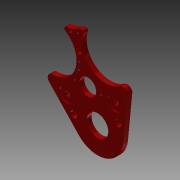
# Autodesk Inventor part: OutlineSketch1
Saved by Autodesk Inventor 2013 (Build 170138000, 138)
## iProperties
Created: 2013-06-03
Part Number: OutlineSketch1
Material: Aluminum 6061
Document SubType Name: Modeling
Designer: mvarma
Density: 2.71 g/cm^3
Mass: 149.846 g
Surface Area: 274.597 cm^2
Volume: 55.2937 cm^3
Author: mvarma
Autodesk Inventor part; units mm, degrees
ref_plane "YZ Plane" through (0, 0, 0) normal (1, 0, 0) x (0, 1, 0)
ref_plane "XZ Plane" through (0, 0, 0) normal (0, 1, 0) x (-1, 0, 0)
ref_plane "XY Plane" through (0, 0, 0) normal (0, 0, 1) x (1, 0, 0)
sketch "Sketch1" plane through (0, 0, 0) normal (0, 0, 1) x (1, 0, 0)
  line L0 (0, 0) -> (304.8, 0) construction
  line L1 (304.8, 0) -> (304.8, 50.8) construction
  line L2 (304.8, 50.8) -> (0, 50.8) construction
  line L3 (0, 50.8) -> (0, 0) construction
  circle A0 centre (152.4, 23.8125) radius 14.2875
  arc A1 (186.526662, 20.469591) -> (127.726757, 0) centre (152.4, 23.8125) ccw
  circle A2 centre (152.4, 23.8125) radius 26.035 construction
  line L4 (152.4, 23.8125) -> (139.519977, 61.741013) construction
  circle A3 centre (139.519977, 61.741013) radius 9.525 construction
  circle A4 centre (139.519977, 61.741013) radius 17.78 construction
  circle A5 centre (91.561866, 85.09) radius 31.75 construction
  arc A6 (133.1868, 119.400632) -> (182.101149, 83.849872) centre (163.342398, 109.465722) ccw
  circle A7 centre (109.531215, 150.050573) radius 31.75 construction
  line L5 (0, 50.8) -> (0, 53.34) construction
  line L6 (0, 53.34) -> (304.8, 53.34) construction
  line L7 (304.8, 53.34) -> (304.8, 50.8) construction
  circle A8 centre (139.519977, 61.741013) radius 21.59 construction
  circle A9 centre (152.4, 23.8125) radius 46.99 construction
  circle A10 centre (152.4, 23.8125) radius 50.8 construction
  arc A11 (86.386473, 79.456368) -> (92.43632, 92.689857) centre (91.561866, 85.09) ccw construction
  circle A12 centre (163.342398, 109.465722) radius 7.65 construction
  arc A13 (116.774938, 152.510446) -> (102.287492, 147.5907) centre (109.531215, 150.050573) ccw construction
  circle A14 centre (139.519977, 61.741013) radius 22.9 construction
  line L8 (86.386473, 79.456368) -> (124.027623, 44.87694) construction
  line L9 (170.878164, 108.148633) -> (162.078023, 57.798354) construction
  line L10 (92.43632, 92.689857) -> (91.561866, 85.09) construction
  line L11 (91.561866, 85.09) -> (86.386473, 79.456368) construction
  circle A15 centre (127.673753, 96.62524) radius 3.175 construction
  circle A16 centre (127.673753, 96.62524) radius 7.9375 construction
  line L12 (92.43632, 92.689857) -> (126.766436, 88.739767) construction
  line L13 (133.195304, 90.922926) -> (158.02084, 114.961496) construction
  line L14 (158.02084, 114.961496) -> (163.342398, 109.465722) construction
  line L15 (170.878164, 108.148633) -> (163.342398, 109.465722) construction
  line L16 (139.519977, 61.741013) -> (127.673753, 96.62524) construction
  line L17 (91.561866, 85.09) -> (163.342398, 109.465722) construction
  line L18 (152.4, 23.8125) -> (91.561866, 85.09) construction
  line L19 (152.4, 23.8125) -> (163.342398, 109.465722) construction
  circle A17 centre (127.673753, 96.62524) radius 9.2075 construction
  circle A18 centre (127.673753, 96.62524) radius 6.1595 construction
  arc A19 (92.43632, 92.689857) -> (86.386473, 79.456368) centre (91.561866, 85.09) ccw construction
  circle A20 centre (163.342398, 109.465722) radius 25.4 construction
  circle A21 centre (109.531215, 150.050573) radius 25.4 construction
  line L20 (104.762695, 113.965606) -> (78.361037, 56.214394) construction
  circle A22 centre (91.561866, 85.09) radius 25.4 construction
  line L21 (139.595033, 160.25985) -> (79.467396, 139.841297) construction
  circle A23 centre (139.519977, 61.741013) radius 11.1125
  arc A24 (100.13733, 146.057474) -> (119.680223, 151.623238) centre (109.908777, 148.840356) ccw construction
  line L22 (109.093738, 151.240444) -> (85.48016, 141.883152) construction
  line L23 (109.908777, 148.840356) -> (85.48016, 141.883152) construction
  line L24 (109.093738, 151.240444) -> (132.707317, 160.597736) construction
  line L25 (109.908777, 148.840356) -> (134.337393, 155.79756) construction
  arc A25 (134.92109, 161.474983) -> (130.493544, 159.72049) centre (132.707317, 160.597736) ccw construction
  arc A26 (132.04721, 155.145323) -> (136.627576, 156.449798) centre (134.337393, 155.79756) ccw construction
  arc A27 (132.04721, 155.145323) -> (130.493544, 159.72049) centre (85.48016, 141.883152) ccw construction
  arc A28 (136.627576, 156.449798) -> (134.92109, 161.474983) centre (85.48016, 141.883152) ccw construction
  line L26 (132.707317, 160.597736) -> (134.92109, 161.474983) construction
  line L27 (134.337393, 155.79756) -> (136.627576, 156.449798) construction
  arc A29 (119.680223, 151.623238) -> (118.53917, 154.983361) centre (85.48016, 141.883152) ccw construction
  arc A30 (100.13733, 146.057474) -> (99.648307, 147.497527) centre (85.48016, 141.883152) ccw construction
  line L28 (104.40145, 107.079075) -> (92.701327, 84.534295) construction
  line L29 (81.001203, 61.989515) -> (90.396097, 85.588158) construction
  arc A31 (100.671763, 111.399174) -> (98.91022, 106.974429) centre (99.790992, 109.186802) ccw construction
  arc A32 (103.304563, 104.965502) -> (105.498337, 109.192648) centre (104.40145, 107.079075) ccw construction
  arc A33 (103.304563, 104.965502) -> (98.91022, 106.974429) centre (81.001203, 61.989515) ccw construction
  line L30 (99.790992, 109.186802) -> (100.671763, 111.399174) construction
  line L31 (104.40145, 107.079075) -> (105.498337, 109.192648) construction
  arc A34 (105.498337, 109.192648) -> (100.671763, 111.399174) centre (81.001203, 61.989515) ccw construction
  arc A35 (118.53917, 154.983361) -> (99.648307, 147.497527) centre (109.093738, 151.240444) ccw construction
  arc A36 (88.021276, 75.516384) -> (97.381374, 93.552208) centre (92.701327, 84.534295) ccw construction
  line L32 (90.396097, 85.588158) -> (99.790992, 109.186802) construction
  line L33 (92.701327, 84.534295) -> (81.001203, 61.989515) construction
  arc A37 (88.021276, 75.516384) -> (86.63814, 76.148701) centre (81.001203, 61.989515) ccw construction
  arc A38 (97.381374, 93.552208) -> (94.154055, 95.027616) centre (81.001203, 61.989515) ccw construction
  arc A39 (94.154055, 95.027616) -> (86.63814, 76.148701) centre (90.396097, 85.588158) ccw construction
  line L34 (163.342398, 109.465722) -> (140.898549, 121.35831) construction
  line L35 (163.342398, 109.465722) -> (185.786247, 97.573135) construction
  circle A40 centre (139.519977, 61.741013) radius 22.9 construction
  arc A41 (102.287492, 147.5907) -> (116.774938, 152.510446) centre (109.531215, 150.050573) ccw construction
  arc A42 (102.287492, 147.5907) -> (102.622578, 146.765267) centre (109.531215, 150.050573) ccw construction
  circle A43 centre (90.396097, 85.588158) radius 31.75
  arc A44 (107.326481, 112.71527) -> (92.528233, 52.784767) centre (92.701327, 84.534295) ccw
  line L36 (100.671763, 111.399174) -> (102.139715, 115.086462) construction
  line L37 (105.498337, 109.192648) -> (107.326481, 112.71527) construction
  arc A45 (107.326481, 112.71527) -> (102.139715, 115.086462) centre (81.001203, 61.989515) ccw
  circle A46 centre (109.093738, 151.240444) radius 31.75
  arc A47 (120.148005, 118.786726) -> (128.329199, 122.980144) centre (109.908777, 148.840356) ccw
  line L38 (134.92109, 161.474983) -> (138.610711, 162.93706) construction
  line L39 (136.627576, 156.449798) -> (140.444547, 157.536861) construction
  arc A48 (140.444547, 157.536861) -> (138.610711, 162.93706) centre (85.48016, 141.883152) ccw
  line L40 (91.561866, 85.09) -> (109.531215, 150.050573) construction
  line L41 (109.531215, 150.050573) -> (163.342398, 109.465722) construction
  line L42 (139.519977, 61.741013) -> (109.531215, 150.050573) construction
  circle A49 centre (139.519977, 61.741013) radius 17.4625
  line L43 (139.519977, 61.741013) -> (122.057477, 61.741013) construction
  line L44 (139.519977, 61.741013) -> (156.982477, 61.741013) construction
  line L45 (139.519977, 61.741013) -> (156.982477, 61.741013) construction
  circle A50 centre (139.519977, 61.741013) radius 26.71 construction
  circle A51 centre (111.304007, 39.007024) radius 9.525 construction
  circle A52 centre (175.74499, 60.890333) radius 9.525 construction
  line L46 (0, 3.81) -> (304.8, 3.81) construction
  arc A53 (86.506583, 75.488588) -> (95.723262, 93.598122) centre (91.114923, 84.543355) ccw
  arc A54 (92.484334, 95.047874) -> (85.118472, 76.10991) centre (88.801403, 85.578892) ccw
  arc A55 (95.723262, 93.598122) -> (92.484334, 95.047874) centre (79.594076, 61.906436) ccw
  circle A56 centre (120.927752, 20.728389) radius 5.588
  circle A57 centre (179.620141, 39.908401) radius 5.588
  line L47 (152.4, 23.8125) -> (304.8, 25.4) construction
  line L48 (179.620141, 39.908401) -> (152.4, 23.8125) construction
  line L49 (152.4, 23.8125) -> (120.927752, 20.728389) construction
  line L50 (67.343611, 63.755949) -> (87.883117, 42.06842)
  line L51 (186.526662, 20.469591) -> (192.172651, 78.107645)
  arc A58 (109.813264, 111.278343) -> (111.377577, 117.124349) centre (111.524457, 113.952748) ccw
  arc A59 (128.329199, 122.980144) -> (133.1868, 119.400632) centre (130.171241, 120.394123) ccw
  arc A60 (111.377577, 117.124349) -> (120.148005, 118.786726) centre (109.908777, 148.840356) ccw
  arc A61 (128.329199, 122.980144) -> (111.377577, 117.124349) centre (109.908777, 148.840356) ccw
  arc A62 (137.993696, 128.583928) -> (133.1868, 119.400632) centre (163.342398, 109.465722) ccw
  arc A63 (109.813264, 111.278343) -> (107.326481, 112.71527) centre (92.701327, 84.534295) ccw
  arc A64 (92.528233, 52.784767) -> (87.883117, 42.06842) centre (92.493614, 46.434861) ccw
  arc A65 (182.101149, 83.849872) -> (192.172651, 78.107645) centre (185.852899, 78.726702) ccw
  arc A66 (192.172651, 78.107645) -> (182.101149, 83.849872) centre (185.852899, 78.726702) ccw
  arc A67 (97.105346, 50.8) -> (92.528233, 52.784767) centre (92.493614, 46.434861) ccw
  arc A68 (87.883117, 42.06842) -> (97.105346, 50.8) centre (92.493614, 46.434861) ccw
  line L52 (87.883117, 42.06842) -> (127.503315, 0.233714)
  line L53 (192.172651, 78.107645) -> (194.941159, 106.370436)
  arc A69 (182.101149, 83.849872) -> (137.993696, 128.583928) centre (163.342398, 109.465722) ccw
  arc A70 (180.251465, 3.81) -> (186.526662, 20.469591) centre (152.4, 23.8125) ccw
  arc A71 (127.726757, 0) -> (180.251465, 3.81) centre (152.4, 23.8125) ccw
  arc A72 (92.528233, 52.784767) -> (109.813264, 111.278343) centre (92.701327, 84.534295) ccw
  arc A73 (133.1868, 119.400632) -> (128.329199, 122.980144) centre (130.171241, 120.394123) ccw
  arc A74 (111.377577, 117.124349) -> (109.813264, 111.278343) centre (111.524457, 113.952748) ccw
  point P0 (133.582269, 158.217994)
  point P1 (102.122529, 108.190485)
  dimension "d122" = 63.5
  dimension "d1" = 50.8
  dimension "d2" = 28.575
  dimension "d3" = 23.8125
  dimension "d4" = 152.4
  dimension "d7" = 68.58
  dimension "d8" = 52.07
  dimension "d9" = 19.05
  dimension "d10" = 35.56
  dimension "d11" = 40.0558
  dimension "d12" = 63.5
  dimension "d13" = 63.5
  dimension "d14" = 63.5
  dimension "d15" = 2.54
  dimension "d16" = 304.8
  dimension "d17" = 43.18
  dimension "d18" = 93.98
  dimension "d19" = 101.6
  dimension "d21" = 15.3
  dimension "d22" = 15.3
  dimension "d29" = 45.8
  dimension "d30" = 143.991
  dimension "d31" = 6.35
  dimension "d32" = 15.875
  dimension "d33" = 143.991
  dimension "d35" = 18.415
  dimension "d37" = 12.319
  dimension "d40" = 50.8
  dimension "d41" = 50.8
  dimension "d42" = 18.0044
  dimension "d43" = 18.0044
  dimension "d44" = 50.8
  dimension "d57" = 22.225
  dimension "d67" = 25.4
  dimension "d68" = 25.4
  dimension "d69" = 2.86
  dimension "d70" = 25.4
  dimension "d71" = 25.4
  dimension "d72" = 4.7625
  dimension "d75" = 2.86
  dimension "d80" = 4.7625
  dimension "d82" = 4.7625
  dimension "d83" = 50.8
  dimension "d84" = 50.8
  dimension "d85" = 10.16
  dimension "d97" = 48.41875
  dimension "d99" = 20.32
  dimension "d101" = 25.4
  dimension "d102" = 25.4
  dimension "d103" = 10.16
  dimension "d105" = 18.0044
  dimension "d106" = 18.0044
  dimension "d107" = 45.8
  dimension "d109" = 7.65
  dimension "d114" = 63.5
  dimension "d115" = 63.5
  dimension "d116" = 57.15
  dimension "d123" = 63.5
  dimension "d128" = 93.26256
  dimension "d129" = 34.925
  dimension "d130" = 0
  dimension "d138" = 53.42
  dimension "d139" = 19.05
  dimension "d140" = 19.05
  dimension "d154" = 3.81
  constraints: 124 point on circle, 108 end point, 74 centre point, 48 coincident, 43 tangent, 23 point on line, 15 collinear, 8 perpendicular, 3 midpoint, 3 parallel, 2 equal radius, 2 horizontal, 1 equal length, 12 other
  measures "d1" distance of L1.end L0.end
  measures "d2" diameter of A0
  measures "d3" distance from line of L0 A0.centre
  measures "d4" distance from line of L3 A0.centre
  measures "d7" diameter of A1
  measures "d8" diameter of A2
  measures "d9" diameter of A3
  measures "d10" diameter of A4
  measures "d11" distance of L4.start L4.end
  measures "d12" diameter of A5
  measures "d13" diameter of A6
  measures "d14" diameter of A7
  measures "d15" distance of L2.end L5.end
  measures "d16" distance of L0.end L0.start
  measures "d17" diameter of A8
  measures "d18" diameter of A9
  measures "d19" diameter of A10
  measures "d21" diameter of A11
  measures "d22" diameter of A12
  measures "d29" diameter of A14
  measures "d30" angle of L11 L10
  measures "d31" diameter of A15
  measures "d32" diameter of A16
  measures "d33" angle of L15 L14
  measures "d35" diameter of A17
  measures "d37" diameter of A18
  measures "d40" diameter of A20
  measures "d41" diameter of A21
  measures "d42" angle of L10 L20
  measures "d43" angle of L11 L20
  measures "d44" diameter of A22
  measures "d57" diameter of A23
  measures "d67" distance of L22.start L22.end
  measures "d68" distance of L23.start L22.end
  measures "d69" angle of L21 L22
  measures "d70" distance of L22.start L24.end
  measures "d71" distance of L23.start L25.end
  measures "d72" diameter of A25
  measures "d75" angle of L20 L28
  measures "d80" diameter of A31
  measures "d82" diameter of A32
  measures "d83" distance of L29.start L32.end
  measures "d84" distance of L28.start L29.start
  measures "d85" radius of A24
  measures "d97" radius of A33
  measures "d99" diameter of A36
  measures "d101" distance of L29.start L29.end
  measures "d102" distance of L28.end L29.start
  measures "d103" radius of A39
  measures "d105" angle of L34 L14
  measures "d106" angle of L35 L15
  measures "d107" diameter of A40
  measures "d109" radius of A13
  measures "d114" diameter of A43
  measures "d115" diameter of A44
  measures "d116" radius of A45
  measures "d123" diameter of A47
  measures "d128" distance of L42.start L40.end
  measures "d129" diameter of A49
  measures "d130" distance between parallel lines of L45 L44
  measures "d138" diameter of A50
  measures "d139" diameter of A51
  measures "d140" diameter of A52
  measures "d154" distance between parallel lines of L0 L46
sketch "Sketch1 outline for Plates" plane through (0, 0, 0) normal (0, 0, 1) x (1, 0, 0)
  arc A0 (111.377577, 117.124349) -> (109.813264, 111.278343) centre (111.524457, 113.952748) ccw
  arc A1 (109.813264, 111.278343) -> (92.528233, 52.784767) centre (92.701327, 84.534295) cw
  arc A2 (92.528233, 52.784767) -> (87.883117, 42.06842) centre (92.493614, 46.434861) ccw
  line L0 (87.883117, 42.06842) -> (127.503315, 0.233714)
  arc A3 (127.503315, 0.233714) -> (186.526662, 20.469591) centre (152.4, 23.8125) ccw
  line L1 (186.526662, 20.469591) -> (192.172651, 78.107645)
  arc A4 (192.172651, 78.107645) -> (182.101149, 83.849872) centre (185.852899, 78.726702) ccw
  arc A5 (182.101149, 83.849872) -> (133.1868, 119.400632) centre (163.342398, 109.465722) cw
  arc A6 (133.1868, 119.400632) -> (128.329199, 122.980144) centre (130.171241, 120.394123) ccw
  arc A7 (128.329199, 122.980144) -> (111.377577, 117.124349) centre (109.908777, 148.840356) cw
extrude "Plates" add sketch "Sketch1 outline for Plates" along normal blind 6.35
sketch "Sketch1 outline for Bearing Cuts" plane through (0, 0, 0) normal (0, 0, 1) x (1, 0, 0)
  circle A0 centre (139.519977, 61.741013) radius 11.1125
  circle A1 centre (152.4, 23.8125) radius 14.2875
extrude "Bearing Cuts" cut sketch "Sketch1 outline for Bearing Cuts" along normal blind 25.4
hole "Encoder Mounting Holes" at (122.057477, 61.741013, 0) at (156.982477, 61.741013, 0) direction (0, 0, 1) diameter 2.6416 end through all thread size "6-32 UNC" class "2B" standard "ANSI Unified Screw Threads"
hole "10-32 Pem Nut Holes" at (81.001203, 61.989515, 0) at (85.48016, 141.883152, 0) at (100.671763, 111.399174, 0) at (105.498337, 109.192648, 0) at (102.122529, 108.190485, 0) at (127.673753, 96.62524, 0) at (111.304007, 39.007024, 0) at (175.74499, 60.890333, 0) direction (0, 0, 1) diameter 6.35 end through all
hole "1/4-20 Pem Nut Holes" at (185.786247, 97.573135, 0) at (140.898549, 121.35831, 0) at (120.927752, 20.728389, 0) at (179.620141, 39.908401, 0) at (133.582269, 158.217994, 0) direction (0, 0, 1) diameter 8.7376 end through all
sketch "Sketch5" plane through (0, 0, 0) normal (0, 0, -1) x (-1, 0, 0)
  line L0 (-124.451327, 85.236013) -> (-124.451327, 75.711013)
  line L1 (-124.451327, 85.236013) -> (-127.626327, 85.236013)
  line L2 (-127.626327, 85.236013) -> (-127.626327, 75.711013)
  line L3 (-127.626327, 75.711013) -> (-124.451327, 75.711013)
  line L4 (-139.519977, 61.741013) -> (-109.908777, 148.840356) construction
  line L5 (-124.637437, 120.312993) -> (-115.619346, 117.247108) construction
  line L6 (-124.637437, 120.312993) -> (-125.659399, 117.306962) construction
  line L7 (-125.659399, 117.306962) -> (-116.641307, 114.241078) construction
  line L8 (-116.641307, 114.241078) -> (-115.619346, 117.247108) construction
  circle A0 centre (-139.519977, 61.741013) radius 11.1125
  arc A1 (-128.329199, 122.980144) -> (-111.377577, 117.124349) centre (-109.908777, 148.840356) ccw
  arc A2 (-109.813264, 111.278343) -> (-92.528233, 52.784767) centre (-92.701327, 84.534295) ccw
  dimension "d196" = 9.525
  dimension "d198" = 3.175
  dimension "d201" = 13.97
  dimension "d209" = 9.525
  dimension "d210" = 3.175
  constraints: 18 end point, 6 coincident, 5 perpendicular, 2 parallel, 2 tangent, 1 symmetric about line, 1 vertical
  measures "d196" distance of L0.start L0.end
  measures "d198" distance of L0.start L1.end
  measures "d201" vertical distance of L4.start point (-127.626, 75.711)
  measures "d209" distance of L5.start L5.end
  measures "d210" distance of L5.start L6.end
hole "Cim Adjustment Block Holes" at (127.626327, 85.236013, 0) at (127.626327, 75.711013, 0) at (125.659399, 117.306962, 0) at (116.641307, 114.241078, 0) direction (0, 0, 1) diameter 2.6416 end through all thread size "6-32 UNC" class "2B" standard "ANSI Unified Screw Threads"
sketch "Sketch8" plane through (0, 0, 6.35) normal (0, 0, 1) x (1, 0, 0)
  circle A0 centre (111.304007, 39.007024) radius 3.175
  circle A1 centre (175.74499, 60.890333) radius 3.175
  circle A2 centre (111.304007, 39.007024) radius 9.525
  circle A3 centre (175.74499, 60.890333) radius 9.525
  point P0 (0, 0)
  dimension "d235" = 19.05
  dimension "d236" = 19.05
  constraints: 2 centre point, 2 coincident
  measures "d235" diameter of A2
  measures "d236" diameter of A3
extrude "Extrusion5" cut sketch "Sketch8" against normal blind 1.190625
sketch "Sketch9" plane through (0, 0, 0) normal (0, 0, -1) x (-1, 0, 0)
  circle A0 centre (-111.304007, 39.007024) radius 3.175
  circle A1 centre (-175.74499, 60.890333) radius 3.175
  circle A2 centre (-175.74499, 60.890333) radius 9.525
  circle A3 centre (-125.659399, 117.306962) radius 1.3208
  circle A4 centre (-127.626327, 85.236013) radius 1.3208
  circle A5 centre (-127.626327, 75.711013) radius 1.3208
  circle A6 centre (-116.641307, 114.241078) radius 1.3208
  circle A7 centre (-179.620141, 39.908401) radius 4.3688
  circle A8 centre (-120.927752, 20.728389) radius 4.3688
  circle A9 centre (-111.304007, 39.007024) radius 3.175
  circle A10 centre (-127.673753, 96.62524) radius 3.175
  circle A11 centre (-175.74499, 60.890333) radius 3.175
  circle A12 centre (-122.057477, 61.741013) radius 1.3208
  circle A13 centre (-156.982477, 61.741013) radius 1.3208
  circle A14 centre (-152.4, 23.8125) radius 14.2875
  circle A15 centre (-139.519977, 61.741013) radius 11.1125
  arc A16 (-182.101149, 83.849872) -> (-192.172651, 78.107645) centre (-185.852899, 78.726702) ccw
  line L0 (-186.526662, 20.469591) -> (-192.172651, 78.107645)
  arc A17 (-186.526662, 20.469591) -> (-127.503315, 0.233714) centre (-152.4, 23.8125) ccw
  line L1 (-87.883117, 42.06842) -> (-127.503315, 0.233714)
  arc A18 (-87.883117, 42.06842) -> (-92.528233, 52.784767) centre (-92.493614, 46.434861) ccw
  arc A19 (-109.813264, 111.278343) -> (-92.528233, 52.784767) centre (-92.701327, 84.534295) ccw
  arc A20 (-109.813264, 111.278343) -> (-111.377577, 117.124349) centre (-111.524457, 113.952748) ccw
  arc A21 (-128.329199, 122.980144) -> (-111.377577, 117.124349) centre (-109.908777, 148.840356) ccw
  arc A22 (-128.329199, 122.980144) -> (-133.1868, 119.400632) centre (-130.171241, 120.394123) ccw
  arc A23 (-182.101149, 83.849872) -> (-133.1868, 119.400632) centre (-163.342398, 109.465722) ccw
  circle A24 centre (-111.304007, 39.007024) radius 9.525
  point P0 (0, 0)
extrude "Extrusion6" cut sketch "Sketch9" against normal blind 1.190625 contours A2 | A24
equation "\"d9\" = Gear15tPD"
equation "\"d10\" = Gear28tPD"
equation "\"d11\" = 0.5 * Gear48tPD + 0.5 * Gear15tPD + MeshingClearance"
equation "\"d12\" = CimOD"
equation "\"d13\" = CimOD"
equation "\"d14\" = CimOD"
equation "\"d17\" = Gear28tPD + ClearanceDiameter"
equation "\"d18\" = WheelOD"
equation "\"d19\" = WheelClearance"
equation "\"Pulley48tPD\" = 45.8"
equation "\"Pulley19tPD\" = 18.2"
equation "\"Pulley16tPD\" = 15.3"
equation "\"Gear15tPD\" = 19.05"
equation "\"Gear35tPD\" = 44.45"
equation "\"Gear48tPD\" = 60.96"
equation "\"Gear28tPD\" = 35.56"
equation "\"BearingLargeOD\" = 28.575"
equation "\"BearingSmallOD\" = 22.225"
equation "\"MeshingClearance\" = 0.0508"
equation "\"CimOD\" = 63.5"
equation "\"WheelOD\" = 93.98"
equation "\"ClearanceDiameter\" = 7.62"
equation "\"WheelClearance\" = 101.6"
equation "\"TensioningBearingID\" = 6.35"
equation "\"TensioningBearingOD\" = 15.875"
equation "\"SpingClipClearance\" = 8.89"
equation "\"Pi\" = 79.79645"
equation "\"Pulley56tPD\" = 53.5"
equation "\"BearingXLargeOD\" = 34.925"
body "Solid3"
